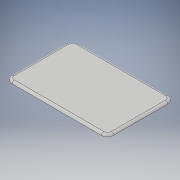
# Autodesk Inventor part: lid-v2
Saved by Autodesk Inventor 2019 (Build 230136000, 136)
## iProperties
Created: 2019-05-24
Part Number: lid-v2
Material: Generic
Document SubType Name: Modeling
Designer: sb002
Density: 1 g/cm^3
Appearance: Default
Author: sb002
## iProperties of the stored document lid-v2_3DPrint.ipt
Created: 2019-05-24
Part Number: lid-v2_3DPrint
Material: Generic
Document SubType Name: Modeling
Designer: sb002
Density: 1 g/cm^3
Appearance: Default
Author: sb002
Autodesk Inventor part; units mm, degrees
ref_plane "YZ Plane" through (0, 0, 0) normal (1, 0, 0) x (0, 1, 0)
ref_plane "XZ Plane" through (0, 0, 0) normal (0, 1, 0) x (-1, 0, 0)
ref_plane "XY Plane" through (0, 0, 0) normal (0, 0, 1) x (1, 0, 0)
sketch "Sketch1" plane through (0, 0, 0) normal (0, 1, 0) x (-1, 0, 0)
  point P0 (0, 0)
sketch "Sketch2" plane through (0, 0, 0) normal (0, 1, 0) x (-1, 0, 0)
  line L0 (6.6745, 14.6831) -> (-112.3255, 14.6831)
  line L1 (-116.3255, 10.6831) -> (-116.3255, -62.3169)
  line L2 (-112.3255, -66.3169) -> (6.6745, -66.3169)
  line L3 (10.6745, -62.3169) -> (10.6745, 10.6831)
  arc A0 (10.6745, 10.6831) -> (6.6745, 14.6831) centre (6.6745, 10.6831) ccw
  arc A1 (6.6745, -66.3169) -> (10.6745, -62.3169) centre (6.6745, -62.3169) ccw
  arc A2 (-116.3255, -62.3169) -> (-112.3255, -66.3169) centre (-112.3255, -62.3169) ccw
  arc A3 (-112.3255, 14.6831) -> (-116.3255, 10.6831) centre (-112.3255, 10.6831) ccw
  point P0 (0, 0)
  point P1 (-116.3255, -66.3169)
  point P2 (-116.3255, 14.6831)
  point P3 (10.6745, -66.3169)
  dimension "d0" = 127
  dimension "d1" = 81
  dimension "d2" = 4
  constraints: 8 end point, 8 point on circle, 8 tangent, 6 point on line, 4 centre point, 3 equal radius, 2 parallel, 1 horizontal, 1 perpendicular
  measures "d0" distance of point (10.675, -66.317) point (-116.325, -66.317)
  measures "d1" distance of point (-116.325, -66.317) point (-116.325, 14.683)
  measures "d2" radius of A0
extrude "Extrusion1" add sketch "Sketch2" along normal blind 2
sketch "Sketch3" plane through (0, 2, 0) normal (0, 1, 0) x (1, 0, 0)
  line L0 (-10.6745, 62.3169) -> (-10.6745, -10.6831) projected
  line L1 (-10.6745, -10.6831) -> (-10.6745, -17.6831)
  line L2 (-10.6745, -17.6831) -> (-13.6745, -17.6831)
  line L3 (-5.6745, -17.6831) -> (111.3255, -17.6831)
  line L4 (119.3255, -9.6831) -> (119.3255, 61.3169)
  line L5 (111.3255, 69.3169) -> (-5.6745, 69.3169)
  line L6 (-13.6745, 61.3169) -> (-13.6745, -9.6831)
  arc A0 (-13.6745, -9.6831) -> (-5.6745, -17.6831) centre (-5.6745, -9.6831) ccw
  arc A1 (111.3255, -17.6831) -> (119.3255, -9.6831) centre (111.3255, -9.6831) ccw
  arc A2 (-5.6745, 69.3169) -> (-13.6745, 61.3169) centre (-5.6745, 61.3169) ccw
  arc A3 (119.3255, 61.3169) -> (111.3255, 69.3169) centre (111.3255, 61.3169) ccw
  point P0 (0, 0)
  point P1 (119.3255, 69.3169)
  point P2 (119.3255, -17.6831)
  point P3 (-13.6745, 69.3169)
  dimension "d5" = 7
  dimension "d6" = 3
  dimension "d7" = 133
  dimension "d8" = 87
  dimension "d9" = 8
  dimension "d10" = 8
  constraints: 12 end point, 8 point on circle, 8 point on line, 8 tangent, 4 centre point, 2 equal radius, 2 parallel, 2 perpendicular, 1 horizontal, 1 vertical
  measures "d5" distance of L0.end L1.end
  measures "d6" distance of L1.end L2.end
  measures "d7" distance of point (-13.675, 69.317) point (119.325, 69.317)
  measures "d8" distance of point (119.325, 69.317) point (119.325, -17.683)
  measures "d9" radius of A0
  measures "d10" radius of A2
extrude "Extrusion2" add sketch "Sketch3" along normal blind 3
fillet "Fillet1" radius 3 8 edges at (116.9823, 5, -66.9738) (52.8255, 5, -69.3169) (-11.3314, 5, -66.9738) (-13.6745, 5, -25.8169) (-11.3314, 5, 15.3399) (52.8255, 5, 17.6831) (116.9823, 5, 15.3399) (119.3255, 5, -25.8169)
fillet "Fillet2" radius 1 8 edges at (-9.503, 0, 13.5115) (-10.6745, 0, -25.8169) (-9.503, 0, -65.1453) (52.8255, 0, -66.3169) (115.1539, 0, -65.1453) (116.3255, 0, -25.8169) (115.1539, 0, 13.5115) (52.8255, 0, 14.6831)
body "Solid1"
